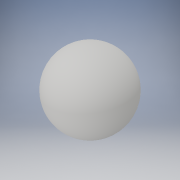
# Autodesk Inventor part: CapBall2
Saved by Autodesk Inventor 2017 (Build 210142000, 142)
## iProperties
Created: 2017-01-28
Part Number: CapBall2
Material: Generic
Document SubType Name: Modeling
Designer: RoboticsUser
Density: 1 g/cm^3
Appearance: Default
Author: RoboticsUser
Autodesk Inventor part; units mm, degrees
ref_plane "YZ Plane" through (0, 0, 0) normal (1, 0, 0) x (0, 1, 0)
ref_plane "XZ Plane" through (0, 0, 0) normal (0, 1, 0) x (-1, 0, 0)
ref_plane "XY Plane" through (0, 0, 0) normal (0, 0, 1) x (1, 0, 0)
sketch "Sketch1" plane through (0, 0, 0) normal (0, 0, 1) x (1, 0, 0)
  circle A0 centre (0, 0) radius 266.7
  dimension "d0" = 533.4
  constraints: 1 centre point, 1 coincident
  measures "d0" diameter of A0
extrude "Extrusion1" add sketch "Sketch1" along normal mid plane 533.4
fillet "Fillet1" radius 266.7 1 edges at (-266.7, 0, 266.7)
sketch "Sketch2" plane through (0, 0, -266.7) normal (0, 0, -1) x (-1, 0, 0)
  point P0 (0, 0)
fillet "Fillet2" radius 266.7 1 edges at (-266.7, 0, -266.7)
body "Solid1"
